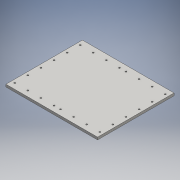
# Autodesk Inventor part: MCPlate2
Saved by Autodesk Inventor 2016 (Build 200138000, 138)
## iProperties
Created: 2015-09-04
Part Number: MCPlate2
Material: Generic
Document SubType Name: Modeling
Designer: Tim
Density: 1 g/cm^3
Appearance: Default
Author: Tim
Autodesk Inventor part; units mm, degrees
ref_plane "YZ Plane" through (0, 0, 0) normal (1, 0, 0) x (0, 1, 0)
ref_plane "XZ Plane" through (0, 0, 0) normal (0, 1, 0) x (-1, 0, 0)
ref_plane "XY Plane" through (0, 0, 0) normal (0, 0, 1) x (1, 0, 0)
sketch "Sketch1" plane through (0, 0, 0) normal (0, 0, 1) x (1, 0, 0)
  line L0 (-112, -93.5) -> (112, -93.5)
  line L1 (112, -93.5) -> (112, 93.5)
  line L2 (112, 93.5) -> (-112, 93.5)
  line L3 (-112, 93.5) -> (-112, -93.5)
  line L4 (-112, -93.5) -> (112, 93.5) construction
  line L5 (112, -93.5) -> (-112, 93.5) construction
  line L6 (-104, -80) -> (104, 80) construction
  line L7 (104, -80) -> (-104, 80) construction
  circle A0 centre (-104, 80) radius 1.85
  circle A1 centre (-104, -80) radius 1.85
  circle A2 centre (104, -80) radius 1.85
  circle A3 centre (104, 80) radius 1.85
  circle A4 centre (-72, 80) radius 1.85 projected
  circle A5 centre (-40, 80) radius 1.85 projected
  circle A6 centre (-8, 80) radius 1.85 projected
  circle A7 centre (8, 80) radius 1.85 projected
  circle A8 centre (40, 80) radius 1.85 projected
  circle A9 centre (72, 80) radius 1.85 projected
  circle A10 centre (-72, -80) radius 1.85 projected
  circle A11 centre (-40, -80) radius 1.85 projected
  circle A12 centre (-8, -80) radius 1.85 projected
  circle A13 centre (8, -80) radius 1.85 projected
  circle A14 centre (40, -80) radius 1.85 projected
  circle A15 centre (72, -80) radius 1.85 projected
  circle A16 centre (104, 48) radius 1.85 projected
  circle A17 centre (104, 16) radius 1.85 projected
  circle A18 centre (104, -16) radius 1.85 projected
  circle A19 centre (104, -48) radius 1.85 projected
  circle A20 centre (-104, -48) radius 1.85 projected
  circle A21 centre (-104, -16) radius 1.85 projected
  circle A22 centre (-104, 16) radius 1.85 projected
  circle A23 centre (-104, 48) radius 1.85 projected
  point P0 (0, 0)
  dimension "d0" = 224
  dimension "d1" = 187
  dimension "d36" = 32
  dimension "d37" = 32
  dimension "d38" = 32
  dimension "d39" = 16
  dimension "d40" = 32
  dimension "d41" = 32
  dimension "d42" = 32
  dimension "d43" = 32
  dimension "d44" = 32
  dimension "d45" = 32
  dimension "d46" = 32
  dimension "d47" = 32
  dimension "d48" = 8
  dimension "d49" = 13.5
  dimension "d50" = 32
  dimension "d51" = 32
  dimension "d52" = 32
  dimension "d53" = 16
  dimension "d54" = 32
  dimension "d55" = 32
  dimension "d56" = 32
  dimension "d57" = 32
  dimension "d58" = 32
  dimension "d59" = 32
  dimension "d60" = 32
  dimension "d61" = 32
  dimension "d62" = 13.5
  dimension "d63" = 8
  dimension "d64" = 8
  dimension "d65" = 13.5
  dimension "d66" = 8
  dimension "d67" = 13.5
  constraints: 16 end point, 4 centre point, 4 coincident, 3 midpoint, 2 parallel, 1 horizontal, 1 perpendicular
  measures "d0" distance of L2.end L1.end
  measures "d1" distance of L1.end L0.end
  measures "d36" distance of A9.centre A8.centre
  measures "d37" distance of A3.centre A9.centre
  measures "d38" distance of A8.centre A7.centre
  measures "d39" distance of A6.centre A7.centre
  measures "d40" distance of A6.centre A5.centre
  measures "d41" distance of A5.centre A4.centre
  measures "d42" distance of A4.centre L7.end
  measures "d43" distance of A23.centre A0.centre
  measures "d44" distance of A22.centre A23.centre
  measures "d45" distance of A22.centre A21.centre
  measures "d46" distance of A20.centre A21.centre
  measures "d47" distance of L6.start A20.centre
  measures "d48" distance from line of L3 A1.centre
  measures "d49" distance from line of L0 L6.start
  measures "d50" distance of A10.centre L6.start
  measures "d51" distance of A11.centre A10.centre
  measures "d52" distance of A12.centre A11.centre
  measures "d53" distance of A13.centre A12.centre
  measures "d54" distance of A13.centre A14.centre
  measures "d55" distance of A15.centre A14.centre
  measures "d56" distance of A15.centre L7.start
  measures "d57" distance of A19.centre L7.start
  measures "d58" distance of A19.centre A18.centre
  measures "d59" distance of A18.centre A17.centre
  measures "d60" distance of A17.centre A16.centre
  measures "d61" distance of A3.centre A16.centre
  measures "d62" distance from line of L2 L7.end
  measures "d63" distance from line of L3 A0.centre
  measures "d64" distance from line of L1 L6.end
  measures "d65" distance from line of L2 L6.end
  measures "d66" distance from line of L1 L7.start
  measures "d67" distance from line of L0 L7.start
extrude "Extrusion9" add sketch "Sketch1" along normal blind 6
body "Solid9"
